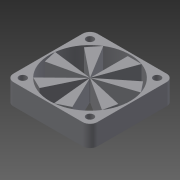
# Autodesk Inventor part: Fan40mm
Saved by Autodesk Inventor 2014 SP1 (Build 180222100, 222)
## iProperties
Created: 2014-02-07
Part Number: Fan40mm
Material: Generic
Document SubType Name: Modeling
Designer: Jack
Density: 1 g/cm^3
Appearance: Default
Author: Jack
Autodesk Inventor part; units mm, degrees
ref_plane "YZ Plane" through (0, 0, 0) normal (1, 0, 0) x (0, 1, 0)
ref_plane "XZ Plane" through (0, 0, 0) normal (0, 1, 0) x (-1, 0, 0)
ref_plane "XY Plane" through (0, 0, 0) normal (0, 0, 1) x (1, 0, 0)
sketch "Sketch1" plane through (0, 0, 0) normal (0, 0, 1) x (1, 0, 0)
  line L0 (0, 0) -> (40, 0)
  line L1 (40, 0) -> (40, 40)
  line L2 (40, 40) -> (0, 40)
  line L3 (0, 40) -> (0, 0)
  dimension "d0" = 40
  dimension "d1" = 40
  constraints: 8 end point, 2 perpendicular, 1 horizontal, 1 parallel
  measures "d0" distance of L0.start L0.end
  measures "d1" distance of L0.end L1.end
extrude "Extrusion1" add sketch "Sketch1" along normal blind 10
hole "Hole1" at (4, 36, 10) direction (0, 0, -1) diameter 3.5 end through all
hole "Hole2" at (4, 4, 10) direction (0, 0, -1) diameter 3.5 end through all
hole "Hole3" at (36, 4, 10) direction (0, 0, -1) diameter 3.5 end through all
hole "Hole4" at (36, 36, 10) direction (0, 0, -1) diameter 3.5 end through all
fillet "Fillet1" radius 3.5 4 edges at (40, 0, 5) (0, 0, 5) (0, 40, 5) (40, 40, 5)
sketch "Sketch2" plane through (0, 0, 10) normal (0, 0, 1) x (1, 0, 0)
  line L0 (36.5, 40) -> (3.5, 40) projected
  line L1 (0, 36.5) -> (0, 3.5) projected
  line L2 (3.5, 0) -> (36.5, 0) projected
  line L3 (40, 3.5) -> (40, 36.5) projected
  line L4 (20, 40) -> (20, 0) construction
  line L5 (0, 20) -> (40, 20) construction
  line L6 (20, 20) -> (20, 38)
  line L7 (20, 20) -> (26.5515, 38)
  line L8 (26.5515, 38) -> (20, 38)
  line L9 (20, 20) -> (5.927, 31.2228)
  line L10 (20, 20) -> (10.0118, 36.345)
  line L11 (10.0118, 36.345) -> (5.927, 31.2228)
  line L12 (20, 20) -> (2.4513, 15.9946)
  line L13 (20, 20) -> (0.9935, 22.3818)
  line L14 (0.9935, 22.3818) -> (2.4513, 15.9946)
  line L15 (20, 20) -> (12.1901, 3.7826)
  line L16 (20, 20) -> (6.2874, 6.6251)
  line L17 (6.2874, 6.6251) -> (12.1901, 3.7826)
  line L18 (20, 20) -> (27.8099, 3.7826)
  line L19 (20, 20) -> (21.9072, 0.94)
  line L20 (21.9072, 0.94) -> (27.8099, 3.7826)
  line L21 (20, 20) -> (37.5487, 15.9946)
  line L22 (20, 20) -> (36.0909, 9.6074)
  line L23 (36.0909, 9.6074) -> (37.5487, 15.9946)
  line L24 (20, 20) -> (34.073, 31.2228)
  line L25 (20, 20) -> (38.1577, 26.1007)
  line L26 (38.1577, 26.1007) -> (34.073, 31.2228)
  circle A0 centre (20, 20) radius 19.1552
  point P0 (0, 0)
  dimension "d41" = 18
  dimension "d42" = 20
  dimension "d45" = 360
  constraints: 46 end point, 5 midpoint, 3 coincident, 1 perpendicular, 1 point on line, 44 other
  measures "d41" distance of L6.start L6.end
  measures "d42" angle of L7 L4
extrude "Extrusion2" cut sketch "Sketch2" against normal blind 10 contours L10 A0 L8 L6 | L13 A0 L11 L9 | L16 A0 L14 L12 | L19 A0 L17 L15 | L22 A0 L20 L18 | L25 A0 L23 L21 | L7 A0 L26 L24
body "Solid1"
